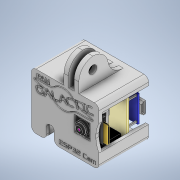
# Autodesk Inventor part: ESP32_cam
Saved by Autodesk Inventor 2022 (Build 260153000, 153)
## iProperties
Created: 2021-10-01
Part Number: ESP32_cam
Material: Generic
Document SubType Name: Modeling
Designer: dech3
Density: 1 g/cm^3
Appearance: Default
Author: dech3
Autodesk Inventor part; units mm, degrees
(part 1 of 4)
ref_plane "YZ Plane" through (0, 0, 0) normal (1, 0, 0) x (0, 1, 0)
ref_plane "XZ Plane" through (0, 0, 0) normal (0, 1, 0) x (-1, 0, 0)
ref_plane "XY Plane" through (0, 0, 0) normal (0, 0, 1) x (1, 0, 0)
sketch "Sketch1" plane through (0, 0, 0) normal (0, 0, 1) x (1, 0, 0)
  line L0 (-17.8, 13.525) -> (17.8, 13.525)
  line L1 (19.8, 11.525) -> (19.8, -11.525)
  line L2 (17.8, -13.525) -> (-17.8, -13.525)
  line L3 (-19.8, -11.525) -> (-19.8, 11.525)
  arc A0 (17.8, -13.525) -> (19.8, -11.525) centre (17.8, -11.525) ccw
  arc A1 (19.8, 11.525) -> (17.8, 13.525) centre (17.8, 11.525) ccw
  arc A2 (-17.8, 13.525) -> (-19.8, 11.525) centre (-17.8, 11.525) ccw
  arc A3 (-19.8, -11.525) -> (-17.8, -13.525) centre (-17.8, -11.525) ccw
  point P0 (0, 0)
  dimension "d0" = 39.6
  dimension "d1" = 27.05
  dimension "d2" = 13.525
  dimension "d3" = 19.8
  dimension "d4" = 2
  constraints: 8 end point, 8 point on circle, 8 tangent, 4 centre point, 3 equal radius, 2 parallel, 1 horizontal, 1 perpendicular
  measures "d0" distance between parallel lines of L1 L3
  measures "d1" distance between parallel lines of L2 L0
  measures "d2" distance from line of point (0, 0) L0
  measures "d3" distance from line of point (0, 0) L1
  measures "d4" radius of A0
extrude "Extrusion1" add sketch "Sketch1" along normal blind 1.6
sketch "Sketch2" plane through (0, 0, 1.6) normal (0, 0, 1) x (1, 0, 0)
  line L0 (4.86, 7.665) -> (19.8, 7.665)
  line L1 (19.8, 7.665) -> (19.8, -7.305)
  line L2 (19.8, -7.305) -> (4.86, -7.305)
  line L3 (4.86, -7.305) -> (4.86, 7.665)
  line L4 (17.8, 13.525) -> (-17.8, 13.525) projected
  line L5 (-17.8, -13.525) -> (17.8, -13.525) projected
  point P0 (0, 0)
  point P1 (19.8, 11.525)
  dimension "d7" = 14.94
  dimension "d8" = 5.86
  dimension "d9" = 6.22
  constraints: 8 end point, 2 parallel, 1 horizontal, 1 perpendicular, 1 vertical alignment
  measures "d7" distance between parallel lines of L1 L3
  measures "d8" distance between parallel lines of L0 L4
  measures "d9" distance between parallel lines of L5 L2
extrude "Extrusion2" add sketch "Sketch2" along normal blind 2 separate body
sketch "Sketch3" plane through (0, 0, 3.6) normal (0, 0, 1) x (1, 0, 0)
  line L0 (7.2, 4.265) -> (15.2, 4.265)
  line L1 (15.2, 4.265) -> (15.2, -3.905)
  line L2 (15.2, -3.905) -> (7.2, -3.905)
  line L3 (7.2, -3.905) -> (7.2, 4.265)
  line L4 (19.8, 7.665) -> (4.86, 7.665) projected
  line L5 (4.86, -7.305) -> (19.8, -7.305) projected
  line L6 (19.8, -7.305) -> (19.8, 7.665) projected
  point P0 (0, 0)
  dimension "d12" = 3.4
  dimension "d13" = 3.4
  dimension "d14" = 4.6
  dimension "d15" = 8
  constraints: 8 end point, 2 parallel, 1 horizontal, 1 perpendicular
  measures "d12" distance between parallel lines of L4 L0
  measures "d13" distance between parallel lines of L5 L2
  measures "d14" distance between parallel lines of L1 L6
  measures "d15" distance between parallel lines of L3 L1
extrude "Extrusion3" add sketch "Sketch3" along normal blind 3.75 separate body
sketch "Sketch4" plane through (0, 0, 7.35) normal (0, 0, 1) x (1, 0, 0)
  circle A0 centre (11.2, 0.18) radius 3.935
  line L0 (15.2, -3.905) -> (15.2, 4.265) projected
  line L1 (7.2, 4.265) -> (7.2, -3.905) projected
  line L2 (15.2, 4.265) -> (7.2, 4.265) projected
  line L3 (7.2, -3.905) -> (15.2, -3.905) projected
  point P0 (0, 0)
  dimension "d18" = 7.87
  dimension "d19" = 8
  dimension "d20" = 4
  dimension "d21" = 4.085
  dimension "d22" = 8.17
  constraints: 1 centre point
  measures "d18" diameter of A0
  measures "d19" distance between parallel lines of L0 L1
  measures "d20" distance from line of L1 A0.centre
  measures "d21" distance from line of L2 A0.centre
  measures "d22" distance between parallel lines of L3 L2
extrude "Extrusion4" add sketch "Sketch4" along normal blind 1.8 contours A0 bodies 3
sketch "Sketch5" plane through (11.2, 0.18, 9.15) normal (0, 0, 1) x (1, 0, 0)
  circle A0 centre (0, 0) radius 3.15
  circle A1 centre (0, 0) radius 3.935 projected
  point P0 (-11.2, -0.18)
  dimension "d25" = 6.3
  constraints: 1 centre point, 1 concentric
  measures "d25" diameter of A0
extrude "Extrusion5" add sketch "Sketch5" along normal blind 1.3 contours A0 bodies 3
sketch "Sketch6" plane through (11.2, 0.18, 10.45) normal (0, 0, 1) x (1, 0, 0)
  circle A0 centre (0, 0) radius 0.85
  circle A1 centre (0, 0) radius 3.15 projected
  point P0 (-11.2, -0.18)
  dimension "d28" = 1.7
  constraints: 1 centre point, 1 concentric
  measures "d28" diameter of A0
extrude "Extrusion6" cut sketch "Sketch6" against normal blind 1 contours A0 bodies 3
chamfer "Chamfer1" distance 1 angle 45 1 edges at (8.05, 0.18, 10.45)
sketch "Sketch7" plane through (11.2, 0.18, 9.45) normal (0, 0, 1) x (1, 0, 0)
  circle A0 centre (0, 0) radius 0.84
  circle A1 centre (0, 0) radius 0.85 projected
  point P0 (-11.2, -0.18)
  dimension "d35" = 0.01
  constraints: 1 centre point, 1 concentric
  measures "d35" radial gap between concentric circles of A1 A0
extrude "Extrusion7" add sketch "Sketch7" along normal blind 1 contours A0 bodies 3
fillet "Fillet2" radius 0.8 1 edges at (10.36, 0.18, 10.45)
sketch "Sketch8" plane through (19.8, -7.305, 1.6) normal (1, 0, 0) x (0, 0, -1)
  line L0 (-0.6, 12.5) -> (-1.8, 12.5)
  line L1 (-1.8, 12.5) -> (-1.8, 0.8)
  line L2 (-1.8, 0.8) -> (-0.6, 0.8)
  line L3 (-0.6, 0.8) -> (-0.6, 12.5)
  line L4 (0, 0) -> (-2, 0) projected
  line L5 (-2, 0) -> (-2, 14.97) projected
  line L6 (0, 14.97) -> (-2, 14.97) projected
  point P0 (1.6, 7.305)
  dimension "d39" = 0.8
  dimension "d40" = 0.2
  dimension "d41" = 2.47
  dimension "d42" = 1.2
  constraints: 8 end point, 2 parallel, 1 horizontal, 1 perpendicular
  measures "d39" distance between parallel lines of L4 L2
  measures "d40" distance between parallel lines of L5 L1
  measures "d41" distance between parallel lines of L6 L0
  measures "d42" distance between parallel lines of L3 L1
extrude "Extrusion8" cut sketch "Sketch8" against normal blind 12 bodies 2
sketch "Sketch9" plane through (7.8, -7.305, 1.6) normal (1, 0, 0) x (0, 0, -1)
  line L0 (-1.7, 12.16) -> (-0.7, 12.16)
  line L1 (-0.7, 12.16) -> (-0.7, 1.14)
  line L2 (-0.7, 1.14) -> (-1.7, 1.14)
  line L3 (-1.7, 1.14) -> (-1.7, 12.16)
  line L4 (-1.8, 0.8) -> (-1.8, 12.5) projected
  line L5 (-0.6, 0.8) -> (-1.8, 0.8) projected
  line L6 (-1.8, 12.5) -> (-0.6, 12.5) projected
  point P0 (1.6, 7.305)
  dimension "d45" = 11.02
  dimension "d46" = 1
  dimension "d47" = 0.1
  dimension "d48" = 0.34
  dimension "d49" = 0.34
  constraints: 8 end point, 2 parallel, 1 horizontal, 1 perpendicular
  measures "d45" distance between parallel lines of L2 L0
  measures "d46" distance between parallel lines of L1 L3
  measures "d47" distance between parallel lines of L4 L3
  measures "d48" distance between parallel lines of L5 L2
  measures "d49" distance between parallel lines of L6 L0
extrude "Extrusion9" add sketch "Sketch9" along normal blind 15 separate body
fillet "Fillet3" radius 0.5 2 edges at (22.8, 4.855, 2.8) (22.8, -6.165, 2.8)
sketch "Sketch10" plane through (0, 0, 0) normal (0, 0, -1) x (-1, 0, 0)
  line L0 (-16.4, 12.525) -> (4.08, 12.525)
  line L1 (4.08, 12.525) -> (4.08, 10.145)
  line L2 (4.08, 10.145) -> (-16.4, 10.145)
  line L3 (-16.4, 10.145) -> (-16.4, 12.525)
  line L4 (-16.4, -10.095) -> (4.08, -10.095)
  line L5 (4.08, -10.095) -> (4.08, -12.475)
  line L6 (4.08, -12.475) -> (-16.4, -12.475)
  line L7 (-16.4, -12.475) -> (-16.4, -10.095)
  line L8 (-17.8, 13.525) -> (17.8, 13.525) projected
  line L9 (17.8, -13.525) -> (-17.8, -13.525) projected
  line L10 (-19.8, -11.525) -> (-19.8, 11.525) projected
  line L11 (19.8, 11.525) -> (19.8, -11.525) projected
  point P0 (0, 0)
  point P1 (-16.4, 11.335)
  point P2 (-16.4, -11.285)
  point P3 (4.08, -11.285)
  point P4 (4.08, 11.335)
  dimension "d53" = 2.38
  dimension "d54" = 2.38
  dimension "d55" = 20.24
  dimension "d56" = 1
  dimension "d57" = 1.05
  dimension "d58" = 3.4
  dimension "d59" = 15.72
  constraints: 16 end point, 4 midpoint, 4 parallel, 2 horizontal, 2 perpendicular, 2 vertical alignment, 1 point on line
  measures "d53" distance between parallel lines of L2 L0
  measures "d54" distance between parallel lines of L6 L4
  measures "d55" distance between parallel lines of L4 L2
  measures "d56" distance between parallel lines of L8 L0
  measures "d57" distance between parallel lines of L9 L6
  measures "d58" distance between parallel lines of L10 L3
  measures "d59" distance between parallel lines of L11 L1
extrude "Extrusion10" add sketch "Sketch10" along normal blind 11.67 separate body
sketch "Sketch11" plane through (0, 0, 0) normal (0, 0, -1) x (-1, 0, 0)
  line L0 (-19.1, 6.625) -> (-15, 6.625)
  line L1 (-15, 6.625) -> (-15, 9.585)
  line L2 (-15, 9.585) -> (-19.1, 9.585)
  line L3 (-19.1, 9.585) -> (-19.1, 6.625)
  line L4 (-19.8, -11.525) -> (-19.8, 11.525) projected
  line L5 (-17.8, 13.525) -> (17.8, 13.525) projected
  point P0 (0, 0)
  dimension "d62" = 0.7
  dimension "d63" = 4.8
  dimension "d64" = 3.94
  dimension "d65" = 6.9
  constraints: 8 end point, 2 parallel, 1 horizontal, 1 perpendicular
  measures "d62" distance between parallel lines of L4 L3
  measures "d63" distance between parallel lines of L1 L4
  measures "d64" distance between parallel lines of L5 L2
  measures "d65" distance between parallel lines of L5 L0
extrude "Extrusion11" add sketch "Sketch11" along normal blind 1.3 separate body
sketch "Sketch12" plane through (0, 0, -1.3) normal (0, 0, -1) x (-1, 0, 0)
  circle A0 centre (-17.05, 8.105) radius 0.88
  line L0 (-19.1, 9.585) -> (-19.1, 6.625) projected
  line L1 (-15, 6.625) -> (-15, 9.585) projected
  line L2 (-15, 9.585) -> (-19.1, 9.585) projected
  line L3 (-19.1, 6.625) -> (-15, 6.625) projected
  point P0 (0, 0)
  dimension "d68" = 1.76
  dimension "d69" = 2.05
  dimension "d70" = 4.1
  dimension "d71" = 1.48
  dimension "d72" = 2.96
  constraints: 1 centre point
  measures "d68" diameter of A0
  measures "d69" distance from line of L0 A0.centre
  measures "d70" distance between parallel lines of L1 L0
  measures "d71" distance from line of L2 A0.centre
  measures "d72" distance between parallel lines of L3 L2
extrude "Extrusion12" add sketch "Sketch12" along normal blind 0.3 separate body contours A0
fillet "Fillet4" radius 0.2 1 edges at (17.93, 8.105, -1.6)
sketch "Sketch13" plane through (0, 0, -11.67) normal (0, 0, -1) x (-1, 0, 0)
  line L0 (-19.65, 16.025) -> (19.65, 16.025)
  line L1 (19.65, 16.025) -> (19.65, -16.115)
  line L2 (19.65, -16.115) -> (-19.65, -16.115)
  line L3 (-19.65, -16.115) -> (-19.65, 16.025)
  line L4 (-16.4, -12.475) -> (4.08, -12.475) projected
  line L5 (4.08, 12.525) -> (-16.4, 12.525) projected
  line L6 (19.8, 11.525) -> (19.8, -11.525) projected
  line L7 (-19.8, -11.525) -> (-19.8, 11.525) projected
  point P0 (0, 0)
  dimension "d76" = 39.3
  dimension "d77" = 32.14
  dimension "d78" = 3.64
  dimension "d79" = 3.5
  dimension "d80" = 0.15
  dimension "d81" = 0.15
  constraints: 8 end point, 2 parallel, 1 horizontal, 1 perpendicular
  measures "d76" distance between parallel lines of L1 L3
  measures "d77" distance between parallel lines of L2 L0
  measures "d78" distance between parallel lines of L2 L4
  measures "d79" distance between parallel lines of L0 L5
  measures "d80" distance between parallel lines of L6 L1
  measures "d81" distance between parallel lines of L7 L3
extrude "Extrusion13" add sketch "Sketch13" along normal blind 1.57 separate body
sketch "Sketch14" plane through (0, 0, -13.24) normal (0, 0, -1) x (-1, 0, 0)
  line L0 (2.75, 15.025) -> (19.75, 15.025)
  line L1 (19.75, 15.025) -> (19.75, 12.305)
  line L2 (19.75, 12.305) -> (2.75, 12.305)
  line L3 (2.75, 12.305) -> (2.75, 15.025)
  line L4 (19.65, 16.025) -> (-19.65, 16.025) projected
  line L5 (19.65, -16.115) -> (19.65, 16.025) projected
  point P0 (0, 0)
  point P1 (19.65, 12.305)
  point P2 (19.65, 15.025)
  dimension "d84" = 1
  dimension "d85" = 3.72
  dimension "d86" = 0.1
  dimension "d87" = 17
  constraints: 8 end point, 2 parallel, 1 horizontal, 1 perpendicular
  measures "d84" distance between parallel lines of L4 L0
  measures "d85" distance between parallel lines of L2 L4
  measures "d86" distance between parallel lines of L5 L1
  measures "d87" distance between parallel lines of L3 L1
extrude "Extrusion14" add sketch "Sketch14" along normal blind 11.08 separate body contours L0 L5 L2 L3
sketch "Sketch15" plane through (0, 0, -13.24) normal (0, 0, -1) x (-1, 0, 0)
  line L0 (11.9, -8.765) -> (19.45, -8.765)
  line L1 (19.45, -8.765) -> (19.45, -14.465)
  line L2 (19.45, -14.465) -> (11.9, -14.465)
  line L3 (11.9, -14.465) -> (11.9, -8.765)
  line L4 (-19.65, -16.115) -> (19.65, -16.115) projected
  line L5 (19.65, -16.115) -> (19.65, 16.025) projected
  point P0 (0, 0)
  dimension "d90" = 7.55
  dimension "d91" = 5.7
  dimension "d147" = 1.65
  dimension "d224" = 0.2
  constraints: 8 end point, 2 parallel, 1 horizontal, 1 perpendicular
  measures "d90" distance between parallel lines of L1 L3
  measures "d91" distance between parallel lines of L2 L0
  measures "d147" distance between parallel lines of L4 L2
  measures "d224" distance between parallel lines of L5 L1
extrude "Extrusion15" add sketch "Sketch15" along normal blind 12 separate body
sketch "Sketch16" plane through (0, 0, -13.24) normal (0, 0, -1) x (-1, 0, 0)
  line L0 (-19.25, 9.175) -> (-18.4, 9.175)
  line L1 (-18.4, 9.175) -> (-18.4, 7.195)
  line L2 (-18.4, 8.325) -> (-19.25, 8.325)
  line L3 (-19.25, 8.325) -> (-19.25, 9.175)
  line L4 (-19.25, -5.575) -> (-18.4, -5.575)
  line L5 (-18.4, -5.575) -> (-18.4, -6.425)
  line L6 (-18.4, -6.425) -> (-19.25, -6.425)
  line L7 (-19.25, -6.425) -> (-19.25, -5.575)
  line L8 (4.5, -5.575) -> (5.35, -5.575)
  line L9 (5.35, -5.575) -> (5.35, -6.425)
  line L10 (5.35, -6.425) -> (4.5, -6.425)
  line L11 (4.5, -6.425) -> (4.5, -5.575)
  line L12 (-19.65, 16.025) -> (-19.65, -16.115) projected
  line L13 (19.65, 16.025) -> (-19.65, 16.025) projected
  point P0 (0, 0)
  dimension "d97" = 0.85
  dimension "d98" = 0.85
  dimension "d99" = 0.85
  dimension "d100" = 0.85
  dimension "d101" = 0.85
  dimension "d102" = 0.85
  dimension "d103" = 0.4
  dimension "d104" = 13.9
  dimension "d105" = 6.85
  dimension "d106" = 22.9
  constraints: 24 end point, 4 parallel, 3 perpendicular, 2 horizontal, 2 point on line, 2 vertical alignment, 1 horizontal alignment
  measures "d97" distance between parallel lines of L1 L3
  measures "d98" distance between parallel lines of L2 L0
  measures "d99" distance between parallel lines of L6 L4
  measures "d100" distance between parallel lines of L5 L7
  measures "d101" distance between parallel lines of L10 L8
  measures "d102" distance between parallel lines of L9 L11
  measures "d103" distance between parallel lines of L12 L3
  measures "d104" distance between parallel lines of L4 L2
  measures "d105" distance between parallel lines of L13 L0
  measures "d106" distance between parallel lines of L11 L5
extrude "Extrusion16" add sketch "Sketch16" along normal blind 5.72 separate body
sketch "Sketch17" plane through (0, 0, -18.96) normal (0, 0, -1) x (-1, 0, 0)
  line L0 (8, 9.925) -> (-19.85, 9.925)
  line L1 (-19.85, 9.925) -> (-19.85, -7.125)
  line L2 (-19.85, -7.125) -> (8, -7.125)
  line L3 (8, -7.125) -> (8, 9.925)
  line L4 (-19.25, -6.425) -> (-18.4, -6.425) projected
  line L5 (-19.65, -16.115) -> (19.65, -16.115) projected
  line L6 (19.65, -16.115) -> (19.65, 16.025) projected
  point P0 (0, 0)
  dimension "d109" = 17.05
  dimension "d110" = 0.7
  dimension "d111" = 8.99
  dimension "d112" = 27.85
  dimension "d113" = 11.65
  constraints: 8 end point, 2 parallel, 1 horizontal, 1 perpendicular
  measures "d109" distance between parallel lines of L2 L0
  measures "d110" distance between parallel lines of L4 L2
  measures "d111" distance between parallel lines of L5 L2
  measures "d112" distance between parallel lines of L3 L1
  measures "d113" distance between parallel lines of L6 L3
extrude "Extrusion17" add sketch "Sketch17" along normal blind 0.93 separate body
sketch "Sketch18" plane through (0, 0, -19.89) normal (0, 0, -1) x (-1, 0, 0)
  line L0 (-21.15, 5.16) -> (-15.71, 5.16)
  line L1 (-15.71, 5.16) -> (-15.71, -2.36)
  line L2 (-15.71, -2.36) -> (-21.15, -2.36)
  line L3 (-21.15, -2.36) -> (-21.15, 5.16)
  line L4 (-19.85, 9.925) -> (-19.85, -7.125) projected
  line L5 (8, 9.925) -> (-19.85, 9.925) projected
  line L6 (-19.85, -7.125) -> (8, -7.125) projected
  point P0 (0, 0)
  dimension "d116" = 7.52
  dimension "d117" = 5.44
  dimension "d118" = 1.3
  dimension "d119" = 4.765
  dimension "d120" = 4.765
  constraints: 8 end point, 2 parallel, 1 horizontal, 1 perpendicular
  measures "d116" distance between parallel lines of L2 L0
  measures "d117" distance between parallel lines of L1 L3
  measures "d118" distance between parallel lines of L4 L3
  measures "d119" distance between parallel lines of L5 L0
  measures "d120" distance between parallel lines of L6 L2
extrude "Extrusion18" add sketch "Sketch18" along normal blind 2.79 separate body
sketch "Sketch19" plane through (21.15, -2.36, -19.89) normal (1, 0, 0) x (0, 0, -1)
  line L0 (0, 6.47) -> (1.39, 7.52)
  line L1 (0, 7.52) -> (2.79, 7.52) projected
  line L2 (1.39, 7.52) -> (0, 7.52)
  line L3 (0, 7.52) -> (0, 6.47)
  line L4 (0, 1.05) -> (1.395, 0)
  line L5 (1.395, 0) -> (0, 0)
  line L6 (0, 0) -> (0, 1.05)
  line L7 (0, 12.285) -> (0, -4.765) projected
  line L8 (2.79, 7.52) -> (2.79, 0) projected
  point P0 (-19.89, 2.36)
  point P1 (1.395, 7.52)
  point P2 (1.39, 7.52)
  dimension "d125" = 5.42
  dimension "d126" = 1.4
  dimension "d127" = 1.05
  dimension "d128" = 1.05
  constraints: 12 end point, 2 collinear, 2 perpendicular, 1 horizontal alignment, 1 midpoint, 1 point on line, 1 vertical alignment
  measures "d125" distance of L4.start L0.start
  measures "d126" distance from line of L8 L0.end
  measures "d127" distance of L1.start L0.start
  measures "d128" distance of L5.end L4.start
extrude "Extrusion19" cut sketch "Sketch19" against normal through all bodies 13
sketch "Sketch20" plane through (21.15, -2.36, -22.68) normal (1, 0, 0) x (0, 0, -1)
  line L0 (-0.4, 7.12) -> (-0.4, 0.4)
  line L1 (-0.4, 0.4) -> (-1.2613, 0.4)
  line L2 (0, 7.52) -> (0, 0) projected
  line L3 (-2.79, 6.47) -> (-2.79, 1.05) projected
  line L4 (-1.4, 7.52) -> (0, 7.52) projected
  line L5 (-1.395, 0) -> (0, 0) projected
  line L6 (-2.39, 6.2709) -> (-1.2659, 7.12)
  line L7 (-2.39, 1.2496) -> (-1.2613, 0.4)
  line L8 (-1.4, 7.52) -> (-2.79, 6.47) projected
  line L9 (-2.79, 1.05) -> (-1.395, 0) projected
  line L10 (-2.39, 1.2496) -> (-2.39, 6.2709)
  line L11 (-1.2659, 7.12) -> (-0.4, 7.12)
  point P0 (-22.68, 2.36)
  dimension "d131" = 0.4
  dimension "d134" = 0.4
  dimension "d135" = 0.4
  dimension "d136" = 0.4
  dimension "d137" = 0.4
  dimension "d138" = 0.4
  constraints: 12 end point, 4 parallel, 1 horizontal, 1 perpendicular
  measures "d131" distance between parallel lines of L2 L0
  measures "d134" distance between parallel lines of L5 L1
  measures "d135" distance between parallel lines of L8 L6
  measures "d136" distance between parallel lines of L9 L7
  measures "d137" distance between parallel lines of L3 L10
  measures "d138" distance between parallel lines of L4 L11
extrude "Extrusion20" cut sketch "Sketch20" against normal blind 5.2375 contours L0 L1 L7 L10 L6 L11 bodies 13
sketch "Sketch21" plane through (0, 0, 1.6) normal (0, 0, 1) x (1, 0, 0)
  line L0 (-11.15, -9.615) -> (-8.15, -9.615)
  line L1 (-8.15, -9.615) -> (-8.15, -12.615)
  line L2 (-8.15, -12.615) -> (-11.15, -12.615)
  line L3 (-11.15, -12.615) -> (-11.15, -9.615)
  line L4 (-19.8, 11.525) -> (-19.8, -11.525) projected
  line L5 (-17.8, -13.525) -> (17.8, -13.525) projected
  point P0 (0, 0)
  dimension "d141" = 3
  dimension "d142" = 3
  dimension "d143" = 8.65
  dimension "d144" = 0.91
  constraints: 8 end point, 2 parallel, 1 horizontal, 1 perpendicular
  measures "d141" distance between parallel lines of L2 L0
  measures "d142" distance between parallel lines of L1 L3
  measures "d143" distance between parallel lines of L4 L3
  measures "d144" distance between parallel lines of L5 L2
extrude "Extrusion21" add sketch "Sketch21" along normal blind 0.85 separate body
sketch "Sketch22" plane through (0, 0, 1.6) normal (0, 0, 1) x (1, 0, 0)
  circle A0 centre (-19.3, 13.025) radius 2.5
  circle A1 centre (19.3, 13.025) radius 2.5
  circle A2 centre (19.3, -13.025) radius 2.5
  circle A3 centre (-19.3, -13.025) radius 2.5
  line L0 (17.8, 13.525) -> (-17.8, 13.525) projected
  line L1 (-19.8, 11.525) -> (-19.8, -11.525) projected
  line L2 (-17.8, -13.525) -> (17.8, -13.525) projected
  line L3 (19.8, -11.525) -> (19.8, 11.525) projected
  point P0 (0, 0)
  dimension "d148" = 5
  dimension "d149" = 5
  dimension "d150" = 5
  dimension "d151" = 5
  dimension "d152" = 0.5
  dimension "d153" = 0.5
  dimension "d154" = 0.5
  dimension "d155" = 0.5
  dimension "d156" = 0.5
  dimension "d157" = 0.5
  dimension "d158" = 0.5
  dimension "d159" = 0.5
  constraints: 4 centre point
  measures "d148" diameter of A0
  measures "d149" diameter of A1
  measures "d150" diameter of A3
  measures "d151" diameter of A2
  measures "d152" distance from line of L0 A0.centre
  measures "d153" distance from line of L1 A0.centre
  measures "d154" distance from line of A3.centre L2
  measures "d155" distance from line of L1 A3.centre
  measures "d156" distance from line of A1.centre L3
  measures "d157" distance from line of L0 A1.centre
  measures "d158" distance from line of L2 A2.centre
  measures "d159" distance from line of L3 A2.centre
extrude "Extrusion22" add sketch "Sketch22" along normal blind 4.5 separate body contours A0 | A1 | A3 | A2
sketch "Sketch23" plane through (19.3, 13.025, 6.1) normal (0, 0, 1) x (1, 0, 0)
  line L0 (-0.5, -31.14) -> (-3.1, -31.14)
  line L1 (-38.1, 5) -> (-0.5, 5)
  line L2 (-28.45, -21.64) -> (-29.45, -21.64)
  line L3 (-4.1, -16.93) -> (-4.1, -8.76) projected
  line L4 (-12.1, -8.76) -> (-12.1, -16.93) projected
  line L5 (-4.1, -8.76) -> (-12.1, -8.76) projected
  line L6 (0.35, -29.14) -> (-38.95, -29.14) projected
  line L7 (-34.45, -31.14) -> (-38.1, -31.14)
  line L8 (-41.1, -28.14) -> (-41.1, 2)
  line L9 (2.5, -31.14) -> (-23.45, -31.14)
  line L10 (-26.45, -28.14) -> (-26.45, -23.64)
  line L11 (-12.1, -16.93) -> (-4.1, -16.93) projected
  line L12 (3.5, -8.67) -> (3.5, -18.69) projected
  line L13 (-38.95, 3) -> (0.35, 3) projected
  line L14 (-13.44, -7.76) -> (-13.44, -17.93)
  line L15 (-39.1, -1.5) -> (-39.1, -24.55) projected
  line L16 (-31.45, -23.64) -> (-31.45, -28.14)
  line L17 (-3.1, -7.76) -> (-13.44, -7.76)
  line L18 (-3.1, -17.93) -> (-3.1, -7.76)
  line L19 (-13.44, -17.93) -> (-3.1, -17.93)
  line L20 (-27.45, -25.64) -> (-27.45, -22.64) projected
  line L21 (-27.45, -22.64) -> (-30.45, -22.64) projected
  line L22 (-30.45, -22.64) -> (-30.45, -25.64) projected
  line L23 (-14.44, -5.36) -> (-14.44, -20.33) projected
  arc A0 (2.5, -5) -> (2.5, -21.64) centre (18.4618, -13.32) ccw
  line L24 (2.5, 2) -> (2.5, -5)
  line L25 (2.5, -21.64) -> (2.5, -28.14)
  line L26 (0.5, -24.55) -> (0.5, -1.5) projected
  arc A1 (-38.1, 5) -> (-41.1, 2) centre (-38.1, 2) ccw
  arc A2 (2.5, 2) -> (-0.5, 5) centre (-0.5, 2) ccw
  arc A3 (-41.1, -28.14) -> (-38.1, -31.14) centre (-38.1, -28.14) ccw
  arc A4 (-34.45, -31.14) -> (-31.45, -28.14) centre (-34.45, -28.14) ccw
  arc A5 (-0.5, -31.14) -> (2.5, -28.14) centre (-0.5, -28.14) ccw
  arc A6 (-29.45, -21.64) -> (-31.45, -23.64) centre (-29.45, -23.64) ccw
  arc A7 (-26.45, -23.64) -> (-28.45, -21.64) centre (-28.45, -23.64) ccw
  arc A8 (-26.45, -28.14) -> (-23.45, -31.14) centre (-23.45, -28.14) ccw
  point P0 (-31.45, -31.14)
  point P1 (-41.1, -31.14)
  point P2 (-26.45, -31.14)
  point P3 (0.5, -12.1472)
  point P4 (0.5, -14.4928)
  dimension "d169" = 2
  dimension "d171" = 2
  dimension "d172" = 1
  dimension "d173" = 1
  dimension "d174" = 1
  dimension "d175" = 2
  dimension "d176" = 1
  dimension "d177" = 1
  dimension "d178" = 1
  dimension "d179" = 1
  dimension "d180" = 9.65
  dimension "d181" = 9.5
  dimension "d182" = 10
  dimension "d183" = 18
  dimension "d184" = 2
  dimension "d185" = 2
  dimension "d186" = 3
  dimension "d187" = 3
  dimension "d188" = 2
  constraints: 28 end point, 18 point on circle, 16 tangent, 9 centre point, 8 point on line, 5 equal radius, 5 parallel, 2 horizontal, 2 horizontal alignment, 1 perpendicular
  measures "d169" distance between parallel lines of L1 L13
  measures "d171" distance between parallel lines of L15 L8
  measures "d172" distance between parallel lines of L10 L20
  measures "d173" distance between parallel lines of L2 L21
  measures "d174" distance between parallel lines of L22 L16
  measures "d175" distance between parallel lines of L6 L9
  measures "d176" distance between parallel lines of L3 L18
  measures "d177" distance between parallel lines of L17 L5
  measures "d178" distance between parallel lines of L23 L14
  measures "d179" distance between parallel lines of L19 L11
  measures "d180" distance of point (-41.1, -31.14) point (-31.45, -31.14)
  measures "d181" distance from line of L0 L25.start
  measures "d182" distance from line of L1 L24.end
  measures "d183" radius of A0
  measures "d184" distance between parallel lines of L26 L25
  measures "d185" distance between parallel lines of L26 L24
  measures "d186" radius of A1
  measures "d187" radius of A5
  measures "d188" radius of A6
extrude "Extrusion23" add sketch "Sketch23" along normal blind 2 contours L0 L9 A8 L10 A7 L2 A6 L16 A4 L7 A3 L8 A1 L1 A2 L24 A0 L25 A5 | A0 L26 bodies 15
sketch "Sketch24" plane through (19.3, 13.025, 6.1) normal (0, 0, -1) x (-1, 0, 0)
  line L0 (41.1, -28.14) -> (41.1, 2)
  line L1 (-0.55, -29.34) -> (-0.55, -21.64)
  line L2 (-0.55, -21.64) -> (-2.5, -21.64)
  line L3 (-2.5, -21.64) -> (-2.5, -28.14)
  line L4 (38.1, 5) -> (0.5, 5)
  line L5 (-0.5, 3.2) -> (39.15, 3.2)
  line L6 (38.95, -29.14) -> (38.95, 3) projected
  line L7 (-0.35, -29.14) -> (38.95, -29.14) projected
  line L8 (38.95, 3) -> (-0.35, 3) projected
  line L9 (-0.35, 3) -> (-0.35, -29.14) projected
  line L10 (-2.5, -26.05) -> (-2.5, -21.64) projected
  line L11 (23.45, -31.14) -> (0.5, -31.14) projected
  line L12 (-2.5, -5) -> (-2.5, 0) projected
  line L13 (0.5, 5) -> (38.1, 5) projected
  line L14 (-2.5, 0) -> (-0.5, 0)
  line L15 (-0.5, 0) -> (-0.5, 3.2)
  line L16 (-0.5, 5) -> (-0.55, 5)
  line L17 (-2.5, 2) -> (-2.5, 0)
  line L18 (41.1, 0) -> (41.1, -26.05) projected
  line L19 (39.15, 3.2) -> (39.15, -29.34)
  arc A0 (38.1, -31.14) -> (41.1, -28.14) centre (38.1, -28.14) ccw
  arc A1 (41.1, 2) -> (38.1, 5) centre (38.1, 2) ccw
  arc A2 (-2.5, -28.14) -> (0.5, -31.14) centre (0.5, -28.14) ccw
  arc A3 (0.5, 5) -> (-2.5, 2) centre (0.5, 2) ccw
  line L20 (31.45, -28.14) -> (31.45, -23.64) projected
  line L21 (26.45, -23.64) -> (26.45, -28.14) projected
  line L22 (39.15, -29.34) -> (31.7005, -29.34)
  line L23 (26.1995, -29.34) -> (-0.55, -29.34)
  line L24 (0.5, -31.14) -> (23.45, -31.14)
  line L25 (34.45, -31.14) -> (38.1, -31.14)
  arc A4 (23.45, -31.14) -> (26.1995, -29.34) centre (23.45, -28.14) ccw
  arc A5 (31.7005, -29.34) -> (34.45, -31.14) centre (34.45, -28.14) ccw
  point P0 (19.3, -13.025)
  point P1 (0.5, -31.14)
  point P2 (23.45, -31.14)
  dimension "d193" = 0.2
  dimension "d194" = 0.2
  dimension "d195" = 0
  dimension "d199" = 0
  dimension "d201" = 0
  dimension "d202" = 0
  dimension "d203" = 2
  dimension "d204" = 0
  dimension "d205" = 3
  dimension "d207" = 0.2
  dimension "d208" = 1.95
  dimension "d211" = 3
  dimension "d212" = 0.2
  dimension "d213" = 3
  dimension "d214" = 1.8
  dimension "d215" = 2.7496
  dimension "d216" = 0.2
  dimension "d217" = 3
  dimension "d218" = 2.7496
  dimension "d219" = 1.8
  dimension "d220" = 66.422
  dimension "d221" = 9.3995
  constraints: 30 end point, 12 point on circle, 12 tangent, 9 parallel, 6 centre point, 4 equal radius, 4 horizontal, 1 perpendicular, 1 point on line
  measures "d193" distance between parallel lines of L8 L5
  measures "d194" distance between parallel lines of L9 L1
  measures "d195" distance between parallel lines of L10 L3
  measures "d199" distance from line of L10.end L2
  measures "d201" distance between parallel lines of L13 L4
  measures "d202" distance between parallel lines of L4 L16
  measures "d203" distance between parallel lines of L17 L15
  measures "d204" distance between parallel lines of L18 L0
  measures "d205" radius of A0
  measures "d207" distance between parallel lines of L6 L19
  measures "d208" distance of L1.end L2.end
  measures "d211" radius of A4
  measures "d212" distance between parallel lines of L7 L23
  measures "d213" radius of A2
  measures "d214" distance between parallel lines of L23 L24
  measures "d215" horizontal distance of L11.start L23.start
  measures "d216" distance between parallel lines of L7 L22
  measures "d217" radius of A5
  measures "d218" horizontal distance of L22.end L25.start
  measures "d219" vertical distance of L22.end L25.start
  measures "d221" distance from line of L0 L22.end
extrude "Extrusion24" add sketch "Sketch24" along normal blind 30 contours A0 L25 A5 L22 L19 L5 L15 L14 L17 A3 L4 A1 L0 | L23 A4 L11 A2 L3 L2 L1 bodies 15
sketch "Sketch26" plane through (19.8, 13.025, 1.6) normal (0, -1, 0) x (1, 0, 0)
  line L0 (0, -14.84) -> (-0.5, -14.84)
  line L1 (-0.5, -14.84) -> (0, -23.84)
  line L2 (0, 0) -> (0, -25.5) projected
  line L3 (0, -23.84) -> (0, -14.84)
  point P0 (-19.8, -1.6)
  point P1 (-0.15, -14.84)
  dimension "d225" = 0.5
  dimension "d226" = 9
  constraints: 6 end point, 2 point on line, 1 coincident, 1 horizontal, 1 horizontal alignment, 1 vertical alignment
  measures "d225" distance from line of L2 L0.end
  measures "d226" distance from line of L1.end L0
extrude "Extrusion25" add sketch "Sketch26" against normal blind 2 bodies 15
sketch "Sketch27" plane through (19.85, -8.615, 6.1) normal (0, 1, 0) x (1, 0, 0)
  line L0 (0.5, 28.34) -> (-0.05, 28.34)
  line L1 (-0.55, 19.34) -> (0.5, 19.34)
  line L2 (0.5, 19.34) -> (0.5, 28.34)
  line L3 (-0.55, 19.34) -> (-0.05, 28.34)
  line L4 (0, 0) -> (0, 30) projected
  point P0 (-19.85, 6.1)
  point P1 (-0.55, 28.34)
  dimension "d229" = 0.5
  constraints: 8 end point, 6 coincident, 1 horizontal, 1 horizontal alignment, 1 parallel
  measures "d229" distance between parallel lines of L2 L4
extrude "Extrusion26" add sketch "Sketch27" against normal blind 2 bodies 15
sketch "Sketch28" plane through (-19.85, -10.5863, 6.1) normal (1, 0, 0) x (0, 0, -1)
  line L0 (28.34, 12.8113) -> (19.34, 12.8113)
  line L1 (19.34, 12.8113) -> (19.34, 14.8113)
  line L2 (19.34, 14.8113) -> (28.34, 14.8113)
  line L3 (28.34, 14.8113) -> (28.34, 12.8113)
  line L4 (0, 26.8113) -> (30, 26.8113) projected
  point P0 (6.1, 10.5863)
  point P1 (19.34, 13.8113)
  point P2 (19.34, 26.6113)
  dimension "d232" = 2
  dimension "d233" = 9
  dimension "d234" = 12
  constraints: 8 end point, 2 parallel, 1 horizontal, 1 midpoint, 1 perpendicular, 1 vertical alignment
  measures "d232" distance between parallel lines of L2 L0
  measures "d233" distance between parallel lines of L3 L1
  measures "d234" distance between parallel lines of L4 L2
extrude "Extrusion27" add sketch "Sketch28" along normal blind 1 bodies 15
chamfer "Chamfer2" distance 9 distance2 1 1 edges at (-18.85, 3.225, -22.24) measured on face at (-18.85, 3.225, -21.74)
sketch "Sketch29" plane through (-18.8, 18.025, 8.1) normal (0, 1, 0) x (1, 0, 0)
  line L0 (18, 19) -> (21, 19)
  line L1 (21, 19) -> (21, 0)
  line L2 (21, 0) -> (18, 0)
  line L3 (18, 0) -> (18, 19)
  line L4 (24.6, 19) -> (27.6, 19)
  line L5 (27.6, 19) -> (27.6, 0)
  line L6 (27.6, 0) -> (24.6, 0)
  line L7 (24.6, 0) -> (24.6, 19)
  line L8 (37.6, 32) -> (37.6, 0) projected
  point P0 (18.8, 8.1)
  dimension "d240" = 19
  dimension "d241" = 3
  dimension "d242" = 3
  dimension "d243" = 3.6
  dimension "d244" = 10
  constraints: 16 end point, 4 parallel, 3 horizontal alignment, 2 horizontal, 2 perpendicular
  measures "d240" distance between parallel lines of L2 L0
  measures "d241" distance between parallel lines of L1 L3
  measures "d242" distance between parallel lines of L5 L7
  measures "d243" distance between parallel lines of L7 L1
  measures "d244" distance between parallel lines of L8 L5
extrude "Extrusion28" add sketch "Sketch29" along normal blind 16.6 bodies 15
sketch "Sketch30" plane through (8.8, 18.025, 8.1) normal (1, 0, 0) x (0, 0, -1)
  circle A0 centre (9, 9) radius 2.625
  line L0 (0, 16.6) -> (19, 16.6) projected
  line L1 (19, 0) -> (19, 16.6) projected
  line L2 (0, 0) -> (0, 16.6) projected
  point P0 (8.1, -18.025)
  dimension "d247" = 5.25
  dimension "d248" = 7.6
  dimension "d249" = 19
  dimension "d250" = 9
  constraints: 1 centre point
  measures "d247" diameter of A0
  measures "d248" distance from line of L0 A0.centre
  measures "d249" distance between parallel lines of L1 L2
  measures "d250" distance from line of L2 A0.centre
extrude "Extrusion29" cut sketch "Sketch30" against normal through all bodies 15
fillet "Fillet5" radius 10 6 edges at (0.7, 34.625, -10.9) (7.3, 34.625, -10.9) (0.7, 34.625, 8.1) (7.3, 34.625, 8.1) (7.3, 18.025, -10.9) (0.7, 18.025, -10.9)
sketch "Sketch31" plane through (19.3, 13.025, 8.1) normal (0, 0, 1) x (1, 0, 0)
  spline S0 degree 3 poles (-34.7908, 1.838) (-34.7811, 1.8603) (-34.7707, 1.8825) (-34.7617, 1.9051) (-34.657, 2.1695) (-34.5593, 2.437) (-34.445, 2.6973) (-34.3859, 2.8319) (-34.3034, 2.9575) (-34.221, 3.0803) (-34.0497, 3.3355) (-33.8154, 3.3203) (-33.6255, 3.1027) (-33.4696, 2.9241) (-33.3348, 2.7243) (-33.2096, 2.5221) (-32.8161, 1.8863) (-32.5037, 1.2122) (-32.2919, 0.4936) (-32.2638, 0.3981) (-32.241, 0.3009) (-32.2212, 0.2033) (-32.21, 0.1483) (-32.1864, 0.1251) (-32.1282, 0.1281) (-32.0075, 0.1343) (-31.9963, 0.0988) (-32.0177, 0.258) (-32.0778, 0.7042) (-32.1395, 1.151) (-32.1742, 1.5996) (-32.2113, 2.0802) (-32.2184, 2.5632) (-32.2385, 3.0452) (-32.2391, 3.0598) (-32.2385, 3.0744) (-32.2386, 3.089) (-32.2392, 3.2024) (-32.216, 3.3044) (-32.0999, 3.3559) (-31.975, 3.4113) (-31.8457, 3.4177) (-31.7442, 3.3196) (-31.5573, 3.1389) (-31.3724, 2.9546) (-31.2035, 2.7573) (-30.9709, 2.4856) (-30.7582, 2.1969) (-30.5281, 1.9228) (-30.4529, 1.8331) (-30.354, 1.7614) (-30.259, 1.691) (-30.1943, 1.6431) (-30.1592, 1.6584) (-30.1499, 1.7382) (-30.1381, 1.8388) (-30.1302, 1.9428) (-30.1424, 2.0428) (-30.1872, 2.4114) (-30.2065, 2.7808) (-30.1887, 3.1515) (-30.1848, 3.2333) (-30.1689, 3.3169) (-30.1436, 3.3948) (-30.098, 3.5348) (-29.9832, 3.5728) (-29.8531, 3.5051) (-29.7387, 3.4455) (-29.684, 3.3414) (-29.6374, 3.2303) (-29.5264, 2.9659) (-29.4686, 2.6879) (-29.4251, 2.4058) (-29.3453, 1.888) (-29.2808, 1.3686) (-29.2691, 0.8441) (-29.2648, 0.6492) (-29.2671, 0.4541) (-29.2694, 0.2591) (-29.2702, 0.197) (-29.2501, 0.1671) (-29.1848, 0.1758) (-28.5603, 0.2591) (-27.9466, 0.383) (-27.3737, 0.659) (-27.0335, 0.8228) (-26.7361, 1.0516) (-26.4366, 1.2773) (-26.0655, 1.5571) (-25.703, 1.8498) (-25.3193, 2.1111) (-24.6979, 2.5344) (-24.0308, 2.8734) (-23.3127, 3.1047) (-22.6944, 3.3037) (-22.0608, 3.4273) (-21.4151, 3.497) (-20.9165, 3.5507) (-20.4167, 3.5553) (-19.9181, 3.5339) (-18.8982, 3.4904) (-17.9119, 3.2844) (-16.9704, 2.8776) (-16.2238, 2.555) (-15.54, 2.1347) (-14.9555, 1.5685) (-14.6238, 1.2471) (-14.3207, 0.896) (-14.0054, 0.5577) (-13.9656, 0.515) (-13.928, 0.4701) (-13.8919, 0.4242) (-13.845, 0.3643) (-13.7861, 0.3525) (-13.716, 0.3715) (-12.7627, 0.6296) (-11.7912, 0.7917) (-10.813, 0.916) (-10.477, 0.9587) (-10.1392, 0.9905) (-9.8, 0.9485) (-9.6279, 0.9271) (-9.4562, 0.9001) (-9.3096, 0.7982) (-9.2045, 0.7252) (-9.1415, 0.6255) (-9.1721, 0.4922) (-9.2026, 0.3592) (-9.297, 0.2867) (-9.4268, 0.2624) (-9.8787, 0.1776) (-10.3313, 0.0968) (-10.7828, 0.0101) (-10.8726, -0.0072) (-10.9599, -0.0407) (-11.0464, -0.0719) (-11.1372, -0.1048) (-11.1793, -0.178) (-11.202, -0.269) (-11.2438, -0.4368) (-11.2023, -0.5985) (-11.1712, -0.7605) (-11.1015, -1.1234) (-11.0295, -1.4858) (-10.9532, -1.8473) (-10.9457, -1.8828) (-10.9084, -1.9273) (-10.8748, -1.9396) (-10.4566, -2.0916) (-10.0419, -2.2568) (-9.6157, -2.3822) (-8.9721, -2.5716) (-8.3199, -2.7319) (-7.6717, -2.9059) (-7.5951, -2.9264) (-7.5555, -2.8808) (-7.5235, -2.8285) (-7.4397, -2.692) (-7.4153, -2.5388) (-7.442, -2.3849) (-7.5081, -2.0041) (-7.582, -1.6246) (-7.6571, -1.2454) (-7.746, -0.7971) (-7.8402, -0.3498) (-7.9309, 0.0982) (-7.9807, 0.3436) (-8.0916, 0.4464) (-8.3387, 0.4678) (-8.4163, 0.4745) (-8.4944, 0.4741) (-8.5722, 0.4792) (-8.6303, 0.483) (-8.6898, 0.4839) (-8.7459, 0.4976) (-8.9235, 0.5409) (-8.992, 0.7175) (-8.8985, 0.8745) (-8.7942, 1.0494) (-8.6225, 1.1165) (-8.4386, 1.1526) (-8.2405, 1.1914) (-8.0393, 1.2145) (-7.8391, 1.2422) (-7.4652, 1.294) (-7.0916, 1.348) (-6.7169, 1.3925) (-6.6023, 1.4061) (-6.4832, 1.401) (-6.3682, 1.3875) (-6.2267, 1.3709) (-6.1216, 1.2721) (-6.1023, 1.1616) (-6.0806, 1.0381) (-6.1476, 0.8994) (-6.2789, 0.8383) (-6.3816, 0.7906) (-6.4934, 0.761) (-6.6033, 0.7308) (-6.8238, 0.6701) (-6.9226, 0.5484) (-6.8975, 0.3204) (-6.8633, 0.0086) (-6.8208, -0.3026) (-6.7684, -0.6118) (-6.6783, -1.144) (-6.5786, -1.6746) (-6.481, -2.2055) (-6.467, -2.2818) (-6.4462, -2.3575) (-6.421, -2.4308) (-6.3423, -2.6595) (-6.1706, -2.751) (-5.9336, -2.7011) (-5.7911, -2.6711) (-5.6477, -2.6422) (-5.5032, -2.6256) (-5.3654, -2.6098) (-5.2355, -2.6427) (-5.1342, -2.7463) (-4.9562, -2.9286) (-5.0397, -3.2467) (-5.2961, -3.3506) (-5.3877, -3.3877) (-5.4863, -3.4076) (-5.5964, -3.4396) (-5.5666, -3.452) (-5.5456, -3.4636) (-5.5231, -3.4696) (-4.46, -3.7519) (-3.4059, -4.0644) (-2.3654, -4.4212) (-2.0639, -4.5246) (-1.761, -4.6318) (-1.5003, -4.8214) (-1.3917, -4.9004) (-1.2877, -4.9957) (-1.209, -5.1036) (-1.0533, -5.3173) (-1.0838, -5.5776) (-1.263, -5.7724) (-1.4413, -5.9664) (-1.6684, -6.0667) (-1.9231, -6.0989) (-2.3941, -6.1586) (-2.8652, -6.2281) (-3.3385, -6.2567) (-4.0167, -6.2976) (-4.697, -6.3272) (-5.3762, -6.3227) (-6.4798, -6.3154) (-7.5831, -6.275) (-8.6866, -6.2514) (-9.3078, -6.2382) (-9.9297, -6.2097) (-10.5503, -6.2255) (-11.385, -6.2468) (-12.2071, -6.3678) (-12.9983, -6.6549) (-13.5047, -6.8387) (-13.9638, -7.1106) (-14.4209, -7.39) (-14.9749, -7.7284) (-15.5263, -8.0734) (-16.098, -8.38) (-16.8167, -8.7655) (-17.5898, -9.0139) (-18.3874, -9.1846) (-19.1584, -9.3496) (-19.9377, -9.4137) (-20.7253, -9.3901) (-21.2696, -9.3737) (-21.8068, -9.3051) (-22.3409, -9.1993) (-22.8994, -9.0886) (-23.4408, -8.9244) (-23.9614, -8.6965) (-24.7827, -8.3369) (-25.5451, -7.8792) (-26.1979, -7.2599) (-26.6165, -6.8628) (-27.0112, -6.4405) (-27.4171, -6.03) (-27.5073, -5.9388) (-27.5995, -5.8496) (-27.6907, -5.7595) (-27.6972, -5.7631) (-27.7038, -5.7666) (-27.7103, -5.7702) (-27.7045, -5.7909) (-27.6981, -5.8114) (-27.6931, -5.8323) (-27.6517, -6.0067) (-27.597, -6.1793) (-27.5727, -6.356) (-27.5432, -6.5712) (-27.7159, -6.7223) (-27.9327, -6.695) (-28.1066, -6.6731) (-28.2563, -6.5942) (-28.4029, -6.5055) (-28.723, -6.312) (-28.988, -6.0549) (-29.2411, -5.7836) (-29.3886, -5.6255) (-29.5283, -5.4582) (-29.6891, -5.3148) (-29.8892, -5.1361) (-30.1284, -5.0394) (-30.4054, -5.0607) (-30.6564, -5.08) (-30.8625, -5.1824) (-31.0209, -5.3798) (-31.16, -5.5532) (-31.2551, -5.7489) (-31.3218, -5.9595) (-31.4388, -6.3288) (-31.6164, -6.6694) (-31.8243, -6.9939) (-31.9164, -7.1375) (-32.0288, -7.2696) (-32.1781, -7.3575) (-32.2423, -7.3953) (-32.3224, -7.4185) (-32.397, -7.4237) (-32.5113, -7.4317) (-32.5926, -7.3729) (-32.6412, -7.2633) (-32.7533, -7.0109) (-32.7522, -6.7457) (-32.7292, -6.4807) (-32.6561, -5.6383) (-32.4383, -4.8295) (-32.1464, -4.0389) (-32.0867, -3.877) (-32.0244, -3.7159) (-31.9579, -3.5566) (-31.9347, -3.5009) (-31.9455, -3.479) (-32.002, -3.4635) (-32.5597, -3.31) (-33.1132, -3.1393) (-33.6753, -3.004) (-34.5429, -2.7951) (-35.4166, -2.6112) (-36.2872, -2.4147) (-36.9812, -2.2582) (-37.6646, -2.0653) (-38.3233, -1.7938) (-38.6564, -1.6565) (-38.9816, -1.5016) (-39.2782, -1.2935) (-39.3873, -1.2169) (-39.48, -1.1241) (-39.5354, -1.0006) (-39.6222, -0.8072) (-39.6072, -0.6192) (-39.4623, -0.4639) (-39.3816, -0.3774) (-39.2771, -0.3041) (-39.17, -0.2526) (-38.7966, -0.0731) (-38.3904, -0.0146) (-37.9851, 0.0411) (-37.8502, 0.0596) (-37.7138, 0.0677) (-37.5779, 0.079) (-37.5311, 0.0828) (-37.5181, 0.0974) (-37.5278, 0.1486) (-37.6076, 0.5737) (-37.6983, 0.9976) (-37.7568, 1.4258) (-37.8162, 1.8607) (-37.8234, 2.3001) (-37.755, 2.737) (-37.7344, 2.8688) (-37.6587, 2.9608) (-37.529, 2.9842) (-37.2061, 3.0425) (-36.8828, 3.1064) (-36.5568, 3.1378) (-36.2765, 3.1648) (-35.9921, 3.1533) (-35.7096, 3.1523) (-35.5311, 3.1516) (-35.3544, 3.13) (-35.1948, 3.0392) (-35.0805, 2.9741) (-35.003, 2.8762) (-34.9516, 2.7566) (-34.862, 2.5478) (-34.8252, 2.3278) (-34.8157, 2.1027) (-34.8121, 2.0169) (-34.8151, 1.9308) (-34.8151, 1.8449) (-34.807, 1.8426) (-34.7989, 1.8403) (-34.7908, 1.838) knots 0 0 0 0 1 1 1 2 2 2 3 3 3 4 4 4 5 5 5 6 6 6 7 7 7 8 8 8 9 9 9 10 10 10 11 11 11 12 12 12 13 13 13 14 14 14 15 15 15 16 16 16 17 17 17 18 18 18 19 19 19 20 20 20 21 21 21 22 22 22 23 23 23 24 24 24 25 25 25 26 26 26 27 27 27 28 28 28 29 29 29 30 30 30 31 31 31 32 32 32 33 33 33 34 34 34 35 35 35 36 36 36 37 37 37 38 38 38 39 39 39 40 40 40 41 41 41 42 42 42 43 43 43 44 44 44 45 45 45 46 46 46 47 47 47 48 48 48 49 49 49 50 50 50 51 51 51 52 52 52 53 53 53 54 54 54 55 55 55 56 56 56 57 57 57 58 58 58 59 59 59 60 60 60 61 61 61 62 62 62 63 63 63 64 64 64 65 65 65 66 66 66 67 67 67 68 68 68 69 69 69 70 70 70 71 71 71 72 72 72 73 73 73 74 74 74 75 75 75 76 76 76 77 77 77 78 78 78 79 79 79 80 80 80 81 81 81 82 82 82 83 83 83 84 84 84 85 85 85 86 86 86 87 87 87 88 88 88 89 89 89 90 90 90 91 91 91 92 92 92 93 93 93 94 94 94 95 95 95 96 96 96 97 97 97 98 98 98 99 99 99 100 100 100 101 101 101 102 102 102 103 103 103 104 104 104 105 105 105 106 106 106 107 107 107 108 108 108 109 109 109 110 110 110 111 111 111 112 112 112 113 113 113 114 114 114 115 115 115 116 116 116 117 117 117 118 118 118 119 119 119 120 120 120 121 121 121 122 122 122 123 123 123 124 124 124 125 125 125 126 126 126 127 127 127 128 128 128 129 129 129 130 130 130 131 131 131 132 132 132 133 133 133 133
  line L0 (-34.7908, 1.838) -> (-34.7811, 1.8603) construction
  line L1 (-34.7811, 1.8603) -> (-34.7707, 1.8825) construction
  line L2 (-34.7707, 1.8825) -> (-34.7617, 1.9051) construction
  line L3 (-34.7617, 1.9051) -> (-34.657, 2.1695) construction
  line L4 (-34.657, 2.1695) -> (-34.5593, 2.437) construction
  line L5 (-34.5593, 2.437) -> (-34.445, 2.6973) construction
  line L6 (-34.445, 2.6973) -> (-34.3859, 2.8319) construction
  line L7 (-34.3859, 2.8319) -> (-34.3034, 2.9575) construction
  line L8 (-34.3034, 2.9575) -> (-34.221, 3.0803) construction
  line L9 (-34.221, 3.0803) -> (-34.0497, 3.3355) construction
  line L10 (-34.0497, 3.3355) -> (-33.8154, 3.3203) construction
  line L11 (-33.8154, 3.3203) -> (-33.6255, 3.1027) construction
  line L12 (-33.6255, 3.1027) -> (-33.4696, 2.9241) construction
  line L13 (-33.4696, 2.9241) -> (-33.3348, 2.7243) construction
  line L14 (-33.3348, 2.7243) -> (-33.2096, 2.5221) construction
  line L15 (-33.2096, 2.5221) -> (-32.8161, 1.8863) construction
  line L16 (-32.8161, 1.8863) -> (-32.5037, 1.2122) construction
  line L17 (-32.5037, 1.2122) -> (-32.2919, 0.4936) construction
  line L18 (-32.2919, 0.4936) -> (-32.2638, 0.3981) construction
  line L19 (-32.2638, 0.3981) -> (-32.241, 0.3009) construction
  line L20 (-32.241, 0.3009) -> (-32.2212, 0.2033) construction
  line L21 (-32.2212, 0.2033) -> (-32.21, 0.1483) construction
  line L22 (-32.21, 0.1483) -> (-32.1864, 0.1251) construction
  line L23 (-32.1864, 0.1251) -> (-32.1282, 0.1281) construction
  line L24 (-32.1282, 0.1281) -> (-32.0075, 0.1343) construction
  line L25 (-32.0075, 0.1343) -> (-31.9963, 0.0988) construction
  line L26 (-31.9963, 0.0988) -> (-32.0177, 0.258) construction
  line L27 (-32.0177, 0.258) -> (-32.0778, 0.7042) construction
  line L28 (-32.0778, 0.7042) -> (-32.1395, 1.151) construction
  line L29 (-32.1395, 1.151) -> (-32.1742, 1.5996) construction
  line L30 (-32.1742, 1.5996) -> (-32.2113, 2.0802) construction
  line L31 (-32.2113, 2.0802) -> (-32.2184, 2.5632) construction
  line L32 (-32.2184, 2.5632) -> (-32.2385, 3.0452) construction
  line L33 (-32.2385, 3.0452) -> (-32.2391, 3.0598) construction
  line L34 (-32.2391, 3.0598) -> (-32.2385, 3.0744) construction
  line L35 (-32.2385, 3.0744) -> (-32.2386, 3.089) construction
  line L36 (-32.2386, 3.089) -> (-32.2392, 3.2024) construction
  line L37 (-32.2392, 3.2024) -> (-32.216, 3.3044) construction
  line L38 (-32.216, 3.3044) -> (-32.0999, 3.3559) construction
  line L39 (-32.0999, 3.3559) -> (-31.975, 3.4113) construction
  line L40 (-31.975, 3.4113) -> (-31.8457, 3.4177) construction
  line L41 (-31.8457, 3.4177) -> (-31.7442, 3.3196) construction
  line L42 (-31.7442, 3.3196) -> (-31.5573, 3.1389) construction
  line L43 (-31.5573, 3.1389) -> (-31.3724, 2.9546) construction
  line L44 (-31.3724, 2.9546) -> (-31.2035, 2.7573) construction
  line L45 (-31.2035, 2.7573) -> (-30.9709, 2.4856) construction
  line L46 (-30.9709, 2.4856) -> (-30.7582, 2.1969) construction
  line L47 (-30.7582, 2.1969) -> (-30.5281, 1.9228) construction
  line L48 (-30.5281, 1.9228) -> (-30.4529, 1.8331) construction
  line L49 (-30.4529, 1.8331) -> (-30.354, 1.7614) construction
  line L50 (-30.354, 1.7614) -> (-30.259, 1.691) construction
  line L51 (-30.259, 1.691) -> (-30.1943, 1.6431) construction
  line L52 (-30.1943, 1.6431) -> (-30.1592, 1.6584) construction
  line L53 (-30.1592, 1.6584) -> (-30.1499, 1.7382) construction
  line L54 (-30.1499, 1.7382) -> (-30.1381, 1.8388) construction
  line L55 (-30.1381, 1.8388) -> (-30.1302, 1.9428) construction
  line L56 (-30.1302, 1.9428) -> (-30.1424, 2.0428) construction
  line L57 (-30.1424, 2.0428) -> (-30.1872, 2.4114) construction
  line L58 (-30.1872, 2.4114) -> (-30.2065, 2.7808) construction
  line L59 (-30.2065, 2.7808) -> (-30.1887, 3.1515) construction
  line L60 (-30.1887, 3.1515) -> (-30.1848, 3.2333) construction
  line L61 (-30.1848, 3.2333) -> (-30.1689, 3.3169) construction
  line L62 (-30.1689, 3.3169) -> (-30.1436, 3.3948) construction
  line L63 (-30.1436, 3.3948) -> (-30.098, 3.5348) construction
  line L64 (-30.098, 3.5348) -> (-29.9832, 3.5728) construction
  line L65 (-29.9832, 3.5728) -> (-29.8531, 3.5051) construction
  line L66 (-29.8531, 3.5051) -> (-29.7387, 3.4455) construction
  line L67 (-29.7387, 3.4455) -> (-29.684, 3.3414) construction
  line L68 (-29.684, 3.3414) -> (-29.6374, 3.2303) construction
  line L69 (-29.6374, 3.2303) -> (-29.5264, 2.9659) construction
  line L70 (-29.5264, 2.9659) -> (-29.4686, 2.6879) construction
  line L71 (-29.4686, 2.6879) -> (-29.4251, 2.4058) construction
  line L72 (-29.4251, 2.4058) -> (-29.3453, 1.888) construction
  line L73 (-29.3453, 1.888) -> (-29.2808, 1.3686) construction
  line L74 (-29.2808, 1.3686) -> (-29.2691, 0.8441) construction
  line L75 (-29.2691, 0.8441) -> (-29.2648, 0.6492) construction
  line L76 (-29.2648, 0.6492) -> (-29.2671, 0.4541) construction
  line L77 (-29.2671, 0.4541) -> (-29.2694, 0.2591) construction
  line L78 (-29.2694, 0.2591) -> (-29.2702, 0.197) construction
  line L79 (-29.2702, 0.197) -> (-29.2501, 0.1671) construction
  line L80 (-29.2501, 0.1671) -> (-29.1848, 0.1758) construction
  line L81 (-29.1848, 0.1758) -> (-28.5603, 0.2591) construction
  line L82 (-28.5603, 0.2591) -> (-27.9466, 0.383) construction
  line L83 (-27.9466, 0.383) -> (-27.3737, 0.659) construction
  line L84 (-27.3737, 0.659) -> (-27.0335, 0.8228) construction
  line L85 (-27.0335, 0.8228) -> (-26.7361, 1.0516) construction
  line L86 (-26.7361, 1.0516) -> (-26.4366, 1.2773) construction
  line L87 (-26.4366, 1.2773) -> (-26.0655, 1.5571) construction
  line L88 (-26.0655, 1.5571) -> (-25.703, 1.8498) construction
  line L89 (-25.703, 1.8498) -> (-25.3193, 2.1111) construction
  line L90 (-25.3193, 2.1111) -> (-24.6979, 2.5344) construction
  line L91 (-24.6979, 2.5344) -> (-24.0308, 2.8734) construction
  line L92 (-24.0308, 2.8734) -> (-23.3127, 3.1047) construction
  line L93 (-23.3127, 3.1047) -> (-22.6944, 3.3037) construction
  line L94 (-22.6944, 3.3037) -> (-22.0608, 3.4273) construction
  line L95 (-22.0608, 3.4273) -> (-21.4151, 3.497) construction
  line L96 (-21.4151, 3.497) -> (-20.9165, 3.5507) construction
  line L97 (-20.9165, 3.5507) -> (-20.4167, 3.5553) construction
  line L98 (-20.4167, 3.5553) -> (-19.9181, 3.5339) construction
  line L99 (-19.9181, 3.5339) -> (-18.8982, 3.4904) construction
  line L100 (-18.8982, 3.4904) -> (-17.9119, 3.2844) construction
  line L101 (-17.9119, 3.2844) -> (-16.9704, 2.8776) construction
  line L102 (-16.9704, 2.8776) -> (-16.2238, 2.555) construction
  line L103 (-16.2238, 2.555) -> (-15.54, 2.1347) construction
  line L104 (-15.54, 2.1347) -> (-14.9555, 1.5685) construction
  line L105 (-14.9555, 1.5685) -> (-14.6238, 1.2471) construction
  line L106 (-14.6238, 1.2471) -> (-14.3207, 0.896) construction
  line L107 (-14.3207, 0.896) -> (-14.0054, 0.5577) construction
  line L108 (-14.0054, 0.5577) -> (-13.9656, 0.515) construction
  line L109 (-13.9656, 0.515) -> (-13.928, 0.4701) construction
  line L110 (-13.928, 0.4701) -> (-13.8919, 0.4242) construction
  line L111 (-13.8919, 0.4242) -> (-13.845, 0.3643) construction
  line L112 (-13.845, 0.3643) -> (-13.7861, 0.3525) construction
  line L113 (-13.7861, 0.3525) -> (-13.716, 0.3715) construction
  line L114 (-13.716, 0.3715) -> (-12.7627, 0.6296) construction
  line L115 (-12.7627, 0.6296) -> (-11.7912, 0.7917) construction
  line L116 (-11.7912, 0.7917) -> (-10.813, 0.916) construction
  line L117 (-10.813, 0.916) -> (-10.477, 0.9587) construction
  line L118 (-10.477, 0.9587) -> (-10.1392, 0.9905) construction
  line L119 (-10.1392, 0.9905) -> (-9.8, 0.9485) construction
  line L120 (-9.8, 0.9485) -> (-9.6279, 0.9271) construction
  line L121 (-9.6279, 0.9271) -> (-9.4562, 0.9001) construction
  line L122 (-9.4562, 0.9001) -> (-9.3096, 0.7982) construction
  line L123 (-9.3096, 0.7982) -> (-9.2045, 0.7252) construction
  line L124 (-9.2045, 0.7252) -> (-9.1415, 0.6255) construction